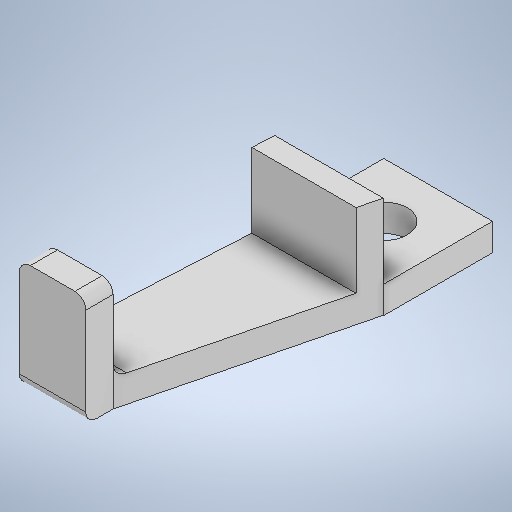
# Autodesk Inventor part: j4 endstop blocker
Saved by Autodesk Inventor 2025 (Build 290162000, 162)
## iProperties
Created: 2025-08-06
Part Number: j4 endstop blocker
Material: 一般
Document SubType Name: Modeling
Designer: gavin
Density: 1 g/cm^3
Appearance: 預設
Author: gavin
## iProperties of the stored document j4 endstop blocker_3D 列印.ipt
Created: 2025-08-06
Part Number: j4 endstop blocker_3D 列印
Material: 一般
Document SubType Name: Modeling
Designer: gavin
Density: 1 g/cm^3
Appearance: 預設
Author: gavin
Autodesk Inventor part; units mm, degrees
ref_plane "XZ Plane" through (0, 0, 0) normal (0, 1, 0) x (-1, 0, 0)
ref_plane "工作平面1" through (-5, 0.8, 4.5) normal (0, -1, 0) x (-1, 0, 0)
sketch "草圖1" plane through (-5, 0.8, 4.5) normal (0, -1, 0) x (-1, 0, 0)
  line L0 (5, 4.5) -> (5, -5.5) projected
  line L1 (-5, 4.5) -> (5, 4.5) projected
  line L2 (-5, -5.5) -> (-5, 4.5) projected
  line L3 (6.1259, -29.105) -> (6.1259, -33.105) construction
  line L4 (6.1259, -29.105) -> (0.026, -29.105) construction
  line L5 (0.026, -33.105) -> (0.026, -29.105) construction
  line L6 (6.1259, -33.105) -> (0.026, -33.105) construction
  line L7 (6.1259, -20.165) -> (6.1259, -24.165) construction
  line L8 (6.1259, -20.165) -> (6.1259, -24.165) construction
  line L9 (6.1259, -20.165) -> (0.026, -20.165) construction
  line L10 (0.026, -24.165) -> (0.026, -20.165) construction
  line L11 (6.1259, -24.165) -> (0.026, -24.165) construction
  line L12 (6.0959, -24.165) -> (6.0959, -29.105) construction
  line L13 (6.0959, -24.165) -> (-0.004, -24.165) construction
  line L14 (-0.004, -29.105) -> (-0.004, -24.165) construction
  line L15 (6.0959, -29.105) -> (-0.004, -29.105) construction
  line L16 (-0.004, -27.885) -> (6.0959, -27.885)
  line L17 (6.0959, -27.885) -> (6.0959, -25.385)
  line L18 (6.0959, -25.385) -> (-0.004, -25.385)
  line L19 (-0.004, -25.385) -> (-0.004, -27.885)
  line L20 (-0.004, -25.385) -> (-5, -5.3334)
  line L21 (6.0959, -25.385) -> (5, -5.3334)
  circle A0 centre (0, -0.5) radius 1.6
  circle A1 centre (0, -0.5) radius 2.165 projected
  line L22 (5, -5.5) -> (-5, -5.5) projected
  point P0 (5, -5.3334)
  point P1 (-4.9585, -5.5)
  dimension "d0" = 2.5
  dimension "d1" = 4.94
  dimension "d2" = 1.22
  dimension "d9" = 3.2
  constraints: 12 end point, 2 parallel, 2 point on line, 1 centre point, 1 horizontal, 1 perpendicular
  measures "d0" distance between parallel lines of L18 L16
  measures "d1" distance between parallel lines of L13 L4
  measures "d2" distance between parallel lines of L4 L16
  measures "d9" diameter of A0
extrude "擠出1" add sketch "草圖1" along normal blind 2.5 contours L0 L22 L20 L2 L1 | L21 L18 L20 L22 L0 | L17 L16 L19 L18 | L20 L22 L2
sketch "草圖2" plane through (-5, 0.8, 4.5) normal (0, 1, 0) x (1, 0, 0)
  line L0 (4.9585, -5.5) -> (0.004, -25.385) projected
  line L1 (5, 4.5) -> (5, -5.5) projected
  line L2 (-5, 4.5) -> (5, 4.5) projected
  line L3 (-5, -5.3334) -> (-5, 4.5) projected
  line L4 (0.004, -25.385) -> (-6.0959, -25.385)
  line L5 (-6.0959, -25.385) -> (-6.0959, -27.885)
  line L6 (-6.0959, -27.885) -> (0.004, -27.885)
  line L7 (0.004, -27.885) -> (0.004, -25.385)
  line L8 (-6.0959, -25.385) -> (-5, -5.3334) projected
  line L9 (-6.0959, -27.885) -> (-6.0959, -25.385) projected
  line L10 (0.004, -27.885) -> (-6.0959, -27.885) projected
  line L11 (0.004, -25.385) -> (0.004, -27.885) projected
  line L12 (5, -5.5) -> (4.9585, -5.5) projected
  constraints: 8 end point, 2 parallel, 1 horizontal, 1 perpendicular
extrude "擠出2" add sketch "草圖2" along normal blind 7.62 contours L7 L6 L5 L4
fillet "圓角1" radius 1 2 edges at (-8.046, 0.8, 29.885) (-8.046, -1.7, 32.385)
fillet "圓角2" radius 1 2 edges at (-4.996, 8.42, 31.135) (-11.0959, 8.42, 31.135)
ref_plane "工作平面2" through (-5, -1.7, 0) normal (1, 0, 0) x (0, 1, 0)
sketch "草圖3" plane through (-5, -1.7, 0) normal (1, 0, 0) x (0, 1, 0)
  line L0 (2.5, 10) -> (2.5, 28.885) projected
  line L1 (0, 10) -> (0, 29.885) projected
  line L2 (2.5, 0) -> (2.5, 10) projected
  line L3 (0, 0) -> (0, 10) projected
  line L4 (2.5, 0) -> (0, 0) projected
  line L5 (2.7, 10) -> (72.85, 10) projected
  line L6 (2.5, 10) -> (9.32, 10)
  line L7 (9.32, 12) -> (2.5, 12)
  line L8 (9.32, 12) -> (9.32, 10)
  arc A0 (3.5, 29.885) -> (2.5, 28.885) centre (3.5, 28.885) ccw projected
  line L9 (3.5, 29.885) -> (0, 29.885) projected
  line L10 (2.5, 10) -> (0, 10) projected
  line L11 (2.5, 10) -> (0, 10) projected
  point P0 (1.7, 0)
  point P1 (9.32, 29.885)
  dimension "d10" = 2
  constraints: 6 end point, 4 point on line, 1 perpendicular, 1 vertical
  measures "d10" distance of L7.start L6.end
extrude "擠出3" add sketch "草圖3" along normal up to surface contours L0 L7 L8 L5 L6 surface through (-0.0415, 0.8, 10) normal (0.9703, 0, 0.2418)
sketch "草圖4" plane through (-5, -1.7, 0) normal (-1, 0, 0) x (0, 0, 1)
  line L0 (12, 9.32) -> (12, 2.5) projected
  line L1 (10, 9.32) -> (12, 9.32) projected
  line L2 (10, 2.5) -> (10, 9.32) projected
  line L3 (12, 2.5) -> (10, 2.5) projected
  point P0 (0, 1.7)
extrude "擠出4" add sketch "草圖4" along normal up to surface surface through (-11.0959, 0.8, 29.885) normal (-0.9985, 0, -0.0546)
